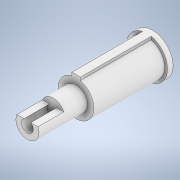
# Autodesk Inventor part: SU22_3DP_EncorderUnit_Bar_sn
Saved by Autodesk Inventor 2022 (Build 260153000, 153)
## iProperties
Created: 2022-06-28
Part Number: SU22_3DP_EncorderUnit_Bar_sn
Material: ABS プラスチック
Document SubType Name: Modeling
Designer: 中島 青蔵
Density: 1.06 g/cm^3
Appearance: 滑らか - 白
Author: 中島 青蔵
Autodesk Inventor part; units mm, degrees
ref_plane "YZ Plane" through (0, 0, 0) normal (1, 0, 0) x (0, 1, 0)
ref_plane "XZ Plane" through (0, 0, 0) normal (0, 1, 0) x (-1, 0, 0)
ref_plane "XY Plane" through (0, 0, 0) normal (0, 0, 1) x (1, 0, 0)
sketch "スケッチ1" plane through (0, 0, 0) normal (0, 0, 1) x (1, 0, 0)
  circle A0 centre (0, 0) radius 7.2
  dimension "d0" = 14.4
  constraints: 1 centre point, 1 coincident
  measures "d0" diameter of A0
extrude "押し出し1" add sketch "スケッチ1" along normal blind 2
sketch "スケッチ2" plane through (0, 0, 2) normal (0, 0, 1) x (1, 0, 0)
  circle A0 centre (0, 0) radius 6.25
  line L0 (-1.5, 6.0673) -> (-1.5, 7.042)
  circle A1 centre (0, 0) radius 7.2 projected
  line L1 (1.5, 7.042) -> (1.5, 6.0673)
  dimension "d3" = 12.5
  dimension "d6" = 1.5
  dimension "d7" = 1.5
  constraints: 4 end point, 4 point on circle, 1 centre point, 1 coincident, 1 parallel, 1 vertical
  measures "d3" diameter of A0
  measures "d6" distance from line of point (0, 0) L1
  measures "d7" distance from line of point (0, 0) L0
extrude "押し出し2" add sketch "スケッチ2" along normal blind 24.8 contours A0 | A0 L0 A1 L1 picked at (1.1681, 6.4463)
sketch "スケッチ3" plane through (0, 0, 26.8) normal (0, 0, 1) x (1, 0, 0)
  circle A0 centre (0, 0) radius 4.05
  circle A1 centre (0, 0) radius 2.05
  line L0 (-1.2, 1.6621) -> (1.2, 1.6621)
  line L1 (-1.2, 1.6621) -> (-3.6932, 1.6621)
  line L2 (1.2, 1.6621) -> (3.6932, 1.6621)
  dimension "d8" = 8.1
  dimension "d9" = 4.1
  dimension "d10" = 2.4
  constraints: 6 end point, 4 point on circle, 2 centre point, 2 coincident, 1 collinear, 1 horizontal, 1 point on line
  measures "d8" diameter of A0
  measures "d9" diameter of A1
  measures "d10" distance of L0.start L0.end
extrude "押し出し3" add sketch "スケッチ3" along normal blind 17 contours A0 L1 A1 L2 picked at (3.3454, -0.3178)
extrude "押し出し4" add sketch "スケッチ3" along normal blind 8 contours L2 A1 L1 A0 | L0 A1 | A1 L0 picked at (-2.7038, 1.9277)
equation "\"d7\" = d6"
